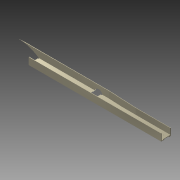
# Autodesk Inventor part: 载板下弹片右
Saved by Autodesk Inventor 2015 (Build 190159000, 159)
## iProperties
Created: 2017-05-16
Part Number: 载板下弹片右
Material: 常规
Document SubType Name: Modeling
Designer: Administrator
Density: 1 g/cm^3
Appearance: 镍
Author: Administrator
Autodesk Inventor part; units mm, degrees
ref_plane "YZ Plane" through (0, 0, 0) normal (1, 0, 0) x (0, 1, 0)
ref_plane "XZ Plane" through (0, 0, 0) normal (0, 1, 0) x (-1, 0, 0)
ref_plane "XY Plane" through (0, 0, 0) normal (0, 0, 1) x (1, 0, 0)
sketch "草图1" plane through (0, 0, 0) normal (0, 0, 1) x (1, 0, 0)
  line L0 (0, 40) -> (-950, 40)
  line L1 (-950, 40) -> (-950, -40)
  line L2 (-950, -40) -> (0, -40)
  line L3 (0, -40) -> (0, 40)
  line L4 (0, 30) -> (-250, 30)
  line L5 (-250, 30) -> (-450, 40)
  point P0 (0, 0)
  point P1 (0, 0)
  dimension "d0" = 950
  dimension "d1" = 80
  dimension "d2" = 250
  dimension "d3" = 200
  dimension "d4" = 10
  constraints: 12 end point, 2 horizontal, 2 parallel, 2 point on line, 1 coincident, 1 midpoint, 1 perpendicular
  measures "d0" distance of L2.end L1.end
  measures "d1" distance of L2.end L0.start
  measures "d2" distance of L4.start L4.end
  measures "d3" horizontal distance of L5.end L4.end
  measures "d4" distance between parallel lines of L0 L4
extrude "拉伸1" add sketch "草图1" along normal blind 50 contours L5 L4 L3 L2 L1 L0
sketch "草图2" plane through (0, -40, 0) normal (1, 0, 0) x (0, 0, -1)
  line L0 (0, 0) -> (0, 70) projected
  line L1 (0, 25) -> (-5, 20)
  line L2 (-5, 20) -> (-5, 60)
  line L3 (-5, 60) -> (0, 55)
  line L4 (0, 0) -> (-50, 0) projected
  line L5 (0, 80) -> (-50, 80) projected
  point P0 (0, 40)
  dimension "d7" = 20
  dimension "d8" = 20
  dimension "d9" = 30
  dimension "d10" = 5
  dimension "d11" = 135
  constraints: 6 end point, 2 point on line, 1 parallel
  measures "d7" distance from line of L4 L1.end
  measures "d8" distance from line of L5 L2.end
  measures "d9" distance of L3.end L1.start
  measures "d10" distance between parallel lines of L0 L2
  measures "d11" angle of L0 L3
extrude "拉伸2" cut sketch "草图2" against normal blind 950
shell "抽壳1" thickness 3 removed faces 3 at (-466.6667, -13.3333, 50) at (0, -10, 35) at (-950, -6.6667, 35)
sketch "草图3" plane through (-950, -27.2426, 8) normal (0, 0, 1) x (1, 0, 0)
  circle A0 centre (925, 27.2426) radius 2.5
  line L0 (0, -12.7574) -> (950, -12.7574) projected
  point P0 (950, 27.2426)
  dimension "d15" = 5
  dimension "d16" = 25
  dimension "d17" = 40
  constraints: 1 centre point
  measures "d15" diameter of A0
  measures "d16" distance of point (950, 27.243) A0.centre
  measures "d17" distance from line of L0 A0.centre
extrude "拉伸3" cut sketch "草图3" against normal blind 3
pattern_linear "矩形阵列1" count 10 spacing 100 along (-1, 0, 0) of "拉伸3"
sketch "草图4" plane through (-950, 40, 0) normal (0, 1, 0) x (1, 0, 0)
  arc A0 (400, 0) -> (450, 0) centre (425, 0) ccw
  line L0 (500, 0) -> (0, 0) projected
  line L1 (950, 0) -> (950, -50) projected
  line L2 (403.3494, -12.5) -> (396.1325, 0)
  line L3 (950, 0) -> (0, 0) projected
  line L4 (446.6506, -12.5) -> (453.8675, 0)
  line L5 (396.1325, 0) -> (453.8675, 0)
  dimension "d23" = 25
  dimension "d24" = 525
  dimension "d25" = 120
  constraints: 6 end point, 4 point on circle, 3 point on line, 2 tangent, 1 centre point, 1 equal length, 1 horizontal, 1 line through centre
  measures "d23" radius of A0
  measures "d24" distance from line of L1 A0.centre
  measures "d25" angle of L0 L4
extrude "拉伸4" cut sketch "草图4" against normal blind 45
sketch "草图5" plane through (-950, 40, 50) normal (0, 1, 0) x (1, 0, 0)
  line L0 (0, 50) -> (0, 0)
  line L1 (0, 0) -> (-150, 0)
  arc A0 (-150, 0) -> (0, 50) centre (-150, 250) ccw
  line L2 (500, 0) -> (0, 0) projected
  point P0 (950, 50)
  dimension "d28" = 150
  constraints: 4 end point, 2 point on circle, 1 centre point, 1 collinear, 1 perpendicular, 1 tangent, 1 vertical
  measures "d28" distance of L0.end L1.end
extrude "拉伸5" add sketch "草图5" against normal blind 3
fillet "圆角1" radius 3 1 edges at (-1020.9431, 40, 37.1708)
